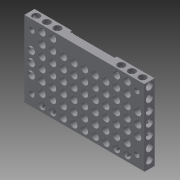
# Autodesk Inventor part: Enclosure-Backplate-Variant02
Saved by Autodesk Inventor 2013 (Build 170138000, 138)
## iProperties
Created: 2014-04-13
Part Number: Enclosure-Backplate-Variant02
Material: Generic
Document SubType Name: Modeling
Designer: spichelh
Density: 1 g/cm^3
Author: spichelh
Autodesk Inventor part; units mm, degrees
ref_plane "YZ Plane" through (0, 0, 0) normal (1, 0, 0) x (0, 1, 0)
sketch "Sketch1" plane through (0, 0, 0) normal (0, 0, 1) x (1, 0, 0)
  line L0 (107.6, 68) -> (107.6, 0)
  line L1 (107.6, 0) -> (0, 0)
  line L2 (0, 0) -> (0, 68)
  line L3 (0, 68) -> (33.75, 68)
  line L4 (33.75, 68) -> (33.75, 61.9)
  line L5 (33.75, 61.9) -> (73.85, 61.9)
  line L6 (73.85, 61.9) -> (73.85, 68)
  line L7 (73.85, 68) -> (107.6, 68)
  line L8 (53.8, 0) -> (53.8, -26.1159) construction
  line L9 (53.8, 61.9) -> (53.8, 35.6829) construction
  dimension "d37" = 40.1
  dimension "d38" = 107.6
  dimension "d39" = 68
  dimension "d64" = 6.1
  constraints: 28 end point, 4 collinear, 3 perpendicular, 2 horizontal, 2 midpoint, 2 parallel, 1 coincident, 1 vertical, 1 other
  measures "d37" distance of L4.end L5.end
  measures "d38" distance of L0.end L1.end
  measures "d39" distance of L1.end L2.end
  measures "d64" distance between parallel lines of L7 L5
extrude "Extrusion1" add sketch "Sketch1" along normal blind 10
sketch "Sketch4" plane through (0, 0, 0) normal (0, 0, -1) x (-1, 0, 0)
  line L0 (-33.75, 68) -> (0, 68) projected
  line L1 (-33.75, 61.9) -> (-33.75, 68) projected
  line L2 (-73.85, 61.9) -> (-33.75, 61.9) projected
  line L3 (-73.85, 68) -> (-73.85, 61.9) projected
  line L4 (-107.6, 68) -> (-73.85, 68) projected
  line L5 (-107.6, 0) -> (-107.6, 68) projected
  line L6 (0, 0) -> (-107.6, 0) projected
  line L7 (0, 68) -> (0, 0) projected
  line L8 (-71.25, 65.4) -> (-71.25, 63.4)
  line L9 (-71.25, 63.4) -> (-36.35, 63.4)
  line L10 (-36.35, 63.4) -> (-36.35, 65.4)
  line L11 (-36.35, 65.4) -> (-2.6, 65.4)
  line L12 (-71.25, 65.4) -> (-105, 65.4)
  line L13 (-105, 65.4) -> (-105, 2.6)
  line L14 (-2.6, 2.6) -> (-2.6, 65.4)
  line L15 (-105, 2.6) -> (-85.29, 2.6)
  line L16 (-85.29, 2.6) -> (-85.29, 5.1)
  line L17 (-85.29, 5.1) -> (-22.31, 5.1)
  line L18 (-22.31, 5.1) -> (-22.31, 2.6)
  line L19 (-22.31, 2.6) -> (-2.6, 2.6)
  line L20 (-53.8, 0) -> (-53.8, 2.6) construction
  line L21 (-53.8, 5.1) -> (-53.8, 2.6) construction
  dimension "d42" = 2.6
  dimension "d43" = 2.6
  dimension "d44" = 2.6
  dimension "d45" = 2.6
  dimension "d46" = 2.6
  dimension "d48" = 2.6
  dimension "d49" = 5.1
  dimension "d50" = 2.6
  dimension "d51" = 2.6
  dimension "d52" = 62.98
  dimension "d65" = 2
  constraints: 28 end point, 6 perpendicular, 4 parallel, 3 collinear, 2 midpoint, 1 horizontal, 1 vertical
  measures "d42" distance between parallel lines of L3 L8
  measures "d43" distance between parallel lines of L1 L10
  measures "d44" distance between parallel lines of L0 L11
  measures "d45" distance between parallel lines of L12 L4
  measures "d46" distance between parallel lines of L5 L13
  measures "d48" distance between parallel lines of L14 L7
  measures "d49" distance between parallel lines of L6 L17
  measures "d50" distance between parallel lines of L6 L15
  measures "d51" distance between parallel lines of L19 L6
  measures "d52" distance between parallel lines of L16 L18
  measures "d65" distance between parallel lines of L12 L9
extrude "Extrusion4" cut sketch "Sketch4" against normal blind 1 contours L0 L7 L6 L5 L4 L3 L12 L13 L15 L16 L17 L18 L19 L14 L11 L1
sketch "Sketch5" plane through (0, 0, 10) normal (0, 0, 1) x (1, 0, 0)
  circle A0 centre (6.8128, 9.8088) radius 1.5 projected
  circle A1 centre (6.81, 59.3388) radius 1.5 projected
  circle A2 centre (100.7928, 9.8142) radius 1.5 projected
  circle A3 centre (100.79, 59.3442) radius 1.5 projected
  line L0 (104.603, 6.0044) -> (3.003, 5.9986) projected
  line L1 (104.5998, 63.1544) -> (104.603, 6.0044) projected
  line L2 (2.9998, 63.1486) -> (104.5998, 63.1544) projected
  line L3 (3.003, 5.9986) -> (2.9998, 63.1486) projected
  circle A4 centre (6.81, 59.3388) radius 1.4
  circle A5 centre (6.8128, 9.8088) radius 1.4
  circle A6 centre (100.7928, 9.8142) radius 1.4
  circle A7 centre (100.79, 59.3442) radius 1.4
  point P0 (0, 0)
  dimension "d55" = 2.8
  dimension "d56" = 2.8
  dimension "d57" = 2.8
  dimension "d58" = 2.8
  constraints: 4 centre point, 4 coincident
  measures "d55" diameter of A4
  measures "d56" diameter of A5
  measures "d57" diameter of A6
  measures "d58" diameter of A7
extrude "Extrusion5" cut sketch "Sketch5" against normal blind 4 contours A4 | A5 | A6 | A7
chamfer "Chamfer3" distance 1 angle 45 4 edges at (5.41, 59.3388, 10) (5.4128, 9.8088, 10) (99.39, 59.3442, 10) (99.3928, 9.8142, 10)
sketch "Sketch6" plane through (33.75, 61.9, 10) normal (1, 0, 0) x (0, 0, -1)
  line L0 (9, 3.5) -> (9, 6.1) projected
  line L1 (10, 0) -> (0, 0) projected
  line L2 (0, 6.1) -> (7, 6.1)
  line L3 (7, 6.1) -> (7, 0)
  line L4 (7, 0) -> (0, 0)
  line L5 (0, 0) -> (0, 6.1)
  point P0 (10, -61.9)
  dimension "d66" = 2
  constraints: 8 end point, 2 parallel, 1 horizontal, 1 perpendicular, 1 point on line
  measures "d66" distance between parallel lines of L3 L0
extrude "Extrusion6" add sketch "Sketch6" along normal blind 41
sketch "Sketch7" plane through (0, 0, 10) normal (0, 0, 1) x (1, 0, 0)
  line L0 (107.6, 68) -> (0, 68) projected
  line L1 (0, 68) -> (0, 0) projected
  line L2 (0, 0) -> (107.6, 0) projected
  line L3 (107.6, 0) -> (107.6, 68) projected
  circle A0 centre (6.175, 62.575) radius 3.175
  circle A1 centre (15.7, 62.575) radius 3.175
  circle A2 centre (25.225, 62.575) radius 3.175
  circle A3 centre (34.75, 62.575) radius 3.175
  circle A4 centre (44.275, 62.575) radius 3.175
  circle A5 centre (53.8, 62.575) radius 3.175
  circle A6 centre (63.325, 62.575) radius 3.175
  circle A7 centre (72.85, 62.575) radius 3.175
  circle A8 centre (82.375, 62.575) radius 3.175
  circle A9 centre (91.9, 62.575) radius 3.175
  circle A10 centre (6.175, 53.05) radius 3.175
  circle A11 centre (15.7, 53.05) radius 3.175
  circle A12 centre (25.225, 53.05) radius 3.175
  circle A13 centre (34.75, 53.05) radius 3.175
  circle A14 centre (44.275, 53.05) radius 3.175
  circle A15 centre (53.8, 53.05) radius 3.175
  circle A16 centre (63.325, 53.05) radius 3.175
  circle A17 centre (72.85, 53.05) radius 3.175
  circle A18 centre (82.375, 53.05) radius 3.175
  circle A19 centre (91.9, 53.05) radius 3.175
  circle A20 centre (6.175, 43.525) radius 3.175
  circle A21 centre (15.7, 43.525) radius 3.175
  circle A22 centre (25.225, 43.525) radius 3.175
  circle A23 centre (34.75, 43.525) radius 3.175
  circle A24 centre (44.275, 43.525) radius 3.175
  circle A25 centre (53.8, 43.525) radius 3.175
  circle A26 centre (63.325, 43.525) radius 3.175
  circle A27 centre (72.85, 43.525) radius 3.175
  circle A28 centre (82.375, 43.525) radius 3.175
  circle A29 centre (91.9, 43.525) radius 3.175
  circle A30 centre (6.175, 34) radius 3.175
  circle A31 centre (15.7, 34) radius 3.175
  circle A32 centre (25.225, 34) radius 3.175
  circle A33 centre (34.75, 34) radius 3.175
  circle A34 centre (44.275, 34) radius 3.175
  circle A35 centre (53.8, 34) radius 3.175
  circle A36 centre (63.325, 34) radius 3.175
  circle A37 centre (72.85, 34) radius 3.175
  circle A38 centre (82.375, 34) radius 3.175
  circle A39 centre (91.9, 34) radius 3.175
  circle A40 centre (6.175, 24.475) radius 3.175
  circle A41 centre (15.7, 24.475) radius 3.175
  circle A42 centre (25.225, 24.475) radius 3.175
  circle A43 centre (34.75, 24.475) radius 3.175
  circle A44 centre (44.275, 24.475) radius 3.175
  circle A45 centre (53.8, 24.475) radius 3.175
  circle A46 centre (63.325, 24.475) radius 3.175
  circle A47 centre (72.85, 24.475) radius 3.175
  circle A48 centre (82.375, 24.475) radius 3.175
  circle A49 centre (91.9, 24.475) radius 3.175
  circle A50 centre (6.175, 14.95) radius 3.175
  circle A51 centre (15.7, 14.95) radius 3.175
  circle A52 centre (25.225, 14.95) radius 3.175
  circle A53 centre (34.75, 14.95) radius 3.175
  circle A54 centre (44.275, 14.95) radius 3.175
  circle A55 centre (53.8, 14.95) radius 3.175
  circle A56 centre (63.325, 14.95) radius 3.175
  circle A57 centre (72.85, 14.95) radius 3.175
  circle A58 centre (82.375, 14.95) radius 3.175
  circle A59 centre (91.9, 14.95) radius 3.175
  circle A60 centre (101.425, 62.575) radius 3.175
  circle A61 centre (101.425, 53.05) radius 3.175
  circle A62 centre (101.425, 43.525) radius 3.175
  circle A63 centre (101.425, 34) radius 3.175
  circle A64 centre (101.425, 24.475) radius 3.175
  circle A65 centre (101.425, 14.95) radius 3.175
  circle A66 centre (6.175, 5.425) radius 3.175
  circle A67 centre (15.7, 5.425) radius 3.175
  circle A68 centre (25.225, 5.425) radius 3.175
  circle A69 centre (34.75, 5.425) radius 3.175
  circle A70 centre (44.275, 5.425) radius 3.175
  circle A71 centre (53.8, 5.425) radius 3.175
  circle A72 centre (63.325, 5.425) radius 3.175
  circle A73 centre (72.85, 5.425) radius 3.175
  circle A74 centre (82.375, 5.425) radius 3.175
  circle A75 centre (91.9, 5.425) radius 3.175
  circle A76 centre (101.425, 5.425) radius 3.175
  dimension "d69" = 6.35
  dimension "d70" = 5.425
  dimension "d71" = 6.175
  dimension "d74" = 9.525
  dimension "d77" = 9.525
  dimension "d80" = 5.425
  dimension "d81" = 6.175
  constraints: 77 centre point, 1 horizontal, 1 vertical, 152 other
  measures "d69" diameter of A0
  measures "d70" distance from line of L0 A0.centre
  measures "d71" distance from line of L1 A0.centre
  measures "d74" distance of A0.centre A1.centre
  measures "d77" distance of A0.centre A10.centre
  measures "d80" distance from line of L2 A66.centre
  measures "d81" distance from line of A62.centre L3
extrude "Extrusion7" cut sketch "Sketch7" against normal blind 7 contours A1 | A2 | A8 | A9 | A11 | A12 | A13 | A14 | A15 | A16 | A17 | A18 | A19 | A20 | A21 | A22 | A23 | A24 | A25 | A26 | A27 | A28 | A29 | A30 | A31 | A32 | A33 | A34 | A35 | A36 | A37 | A38 | A39 | A40 | A41 | A42 | A43 | A44 | A45 | A46 | A47 | A48 | A49 | A51 | A52 | A53 | A54 | A55 | A56 | A57 | A58 | A59 | A62 | A63 | A64 | A67 | A68 | A69 | A70 | A71 | A72 | A73 | A74 | A75
sketch "Sketch8" plane through (0, 68, 10) normal (0, 1, 0) x (1, 0, 0)
  line L0 (0, 9) -> (0, 0) projected
  line L1 (107.6, 0) -> (0, 0) projected
  line L2 (33.75, 9) -> (33.75, 7) projected
  circle A0 centre (15.7, 4.5) radius 3.175
  line L3 (0, 4.5) -> (16.3328, 4.5) construction
  line L4 (18.875, 7) -> (12.525, 7) construction
  line L5 (18.875, 0) -> (12.525, 0) construction
  circle A1 centre (25.225, 4.5) radius 3.175
  line L6 (53.8, 0) -> (53.8, 4.5) construction
  circle A2 centre (91.9, 4.5) radius 3.175
  circle A3 centre (82.375, 4.5) radius 3.175
  circle A4 centre (6.175, 4.5) radius 3.175
  circle A5 centre (101.425, 4.5) radius 3.175
  point P0 (0, 10)
  dimension "d84" = 6.35
  dimension "d85" = 15.7
  dimension "d86" = 12.525
  dimension "d87" = 6.35
  dimension "d88" = 9.525
  dimension "d89" = 6.35
  dimension "d90" = 9.525
  constraints: 6 centre point, 4 end point, 3 point on line, 3 symmetric about line, 2 midpoint, 2 perpendicular, 3 other
  measures "d84" diameter of A0
  measures "d85" distance from line of L0 A0.centre
  measures "d86" distance from line of L0 L4.end
  measures "d87" diameter of A1
  measures "d88" distance of A0.centre A1.centre
  measures "d89" diameter of A4
  measures "d90" distance of A4.centre A0.centre
extrude "Extrusion8" cut sketch "Sketch8" against normal blind 7
ref_plane "Work Plane2" through (0, 34, 10) normal (0, 1, 0) x (1, 0, 0)
mirror "Mirror2" about plane through (0, 34, 10) normal (0, 1, 0) of "Extrusion8"
sketch "Sketch9" plane through (0, 0, 10) normal (-1, 0, 0) x (0, 0, 1)
  line L0 (-9, 0) -> (0, 0) projected
  line L1 (0, 68) -> (0, 0) projected
  line L2 (-9, 68) -> (0, 68) projected
  circle A0 centre (-4.5, 64) radius 3.175
  circle A1 centre (-4.5, 54.475) radius 3.175
  circle A2 centre (-4.5, 44.95) radius 3.175
  circle A3 centre (-4.5, 35.425) radius 3.175
  circle A4 centre (-4.5, 25.9) radius 3.175
  circle A5 centre (-4.5, 16.375) radius 3.175
  circle A6 centre (-4.5, 6.85) radius 3.175
  point P0 (-10, 0)
  dimension "d103" = 10
  dimension "d94" = 6.35
  dimension "d96" = 4.5
  dimension "d97" = 4
  dimension "d100" = 9.525
  dimension "d105" = 6.85
  constraints: 7 centre point, 1 vertical, 12 other
  measures "d94" diameter of A0
  measures "d96" distance from line of A0.centre L1
  measures "d97" distance from line of L2 A0.centre
  measures "d100" distance of A0.centre A1.centre
  measures "d105" distance from line of L0 A6.centre
extrude "Extrusion9" cut sketch "Sketch9" against normal blind 7
ref_plane "Work Plane3" through (53.8, 0, 10) normal (-1, 0, 0) x (0, 0, 1)
mirror "Mirror3" about plane through (53.8, 0, 10) normal (-1, 0, 0) of "Extrusion9"
fillet "Fillet1" radius 0.2 1 edges at (53.8, 68, 10)
fillet "Fillet2" radius 0.2 101 edges at (107.6, 67.9414, 9.9414) (107.6, 33.9, 10) (107.6, 68, 5.4) (0, 67.9414, 9.9414) (0, 68, 5.4) (0, 33.9, 10) (53.8, 0, 10) (22.05, 62.575, 10) (22.05, 53.05, 10) (12.525, 62.575, 10) (12.525, 53.05, 10) (3, 43.525, 10) (12.525, 43.525, 10) (4.41, 59.3388, 10) (3, 68, 5.5) (12.525, 68, 5.5) (22.05, 68, 5.5) (31.575, 53.05, 10) (41.1, 53.05, 10) (50.625, 53.05, 10) (60.15, 53.05, 10) (69.675, 53.05, 10) (79.2, 53.05, 10) (79.2, 62.575, 10) (79.2, 68, 5.5) (88.725, 68, 5.5) (98.25, 68, 5.5) (98.39, 59.3442, 10) (88.725, 53.05, 10) (88.725, 62.575, 10) (88.725, 43.525, 10) (98.25, 43.525, 10) (98.25, 34, 10) (88.725, 34, 10) (79.2, 34, 10) (79.2, 43.525, 10) (69.675, 43.525, 10) (69.675, 34, 10) (60.15, 34, 10) (60.15, 43.525, 10) (50.625, 43.525, 10) (50.625, 34, 10) (41.1, 34, 10) (41.1, 43.525, 10) (31.575, 34, 10) (31.575, 43.525, 10) (22.05, 34, 10) (22.05, 43.525, 10) (12.525, 34, 10) (3, 34, 10) (0, 64, 2.325) (0, 54.475, 2.325) (0, 44.95, 2.325) (0, 35.425, 2.325) (0, 25.9, 2.325) (0, 16.375, 2.325) (0, 6.85, 2.325) (12.525, 5.425, 10) (4.4128, 9.8088, 10) (12.525, 14.95, 10) (12.525, 24.475, 10) (3, 24.475, 10) (22.05, 24.475, 10) (31.575, 24.475, 10) (31.575, 14.95, 10) (22.05, 14.95, 10) (22.05, 5.425, 10) (31.575, 5.425, 10) (41.1, 5.425, 10) (41.1, 14.95, 10) (50.625, 14.95, 10) (50.625, 24.475, 10) (41.1, 24.475, 10) (60.15, 24.475, 10) (60.15, 14.95, 10) (69.675, 14.95, 10) (69.675, 24.475, 10) (79.2, 24.475, 10) (79.2, 14.95, 10) (88.725, 14.95, 10) (88.725, 24.475, 10) (98.25, 24.475, 10) (98.3928, 9.8142, 10) (88.725, 5.425, 10) (79.2, 5.425, 10) (69.675, 5.425, 10) (60.15, 5.425, 10) (50.625, 5.425, 10) (98.25, 0, 5.5) (88.725, 0, 5.5) (79.2, 0, 5.5) (22.05, 0, 5.5) (12.525, 0, 5.5) (3, 0, 5.5) (107.6, 64, 2.325) (107.6, 54.475, 2.325) (107.6, 44.95, 2.325) (107.6, 35.425, 2.325) (107.6, 25.9, 2.325) (107.6, 16.375, 2.325) (107.6, 6.85, 2.325)
body "Solid1"
